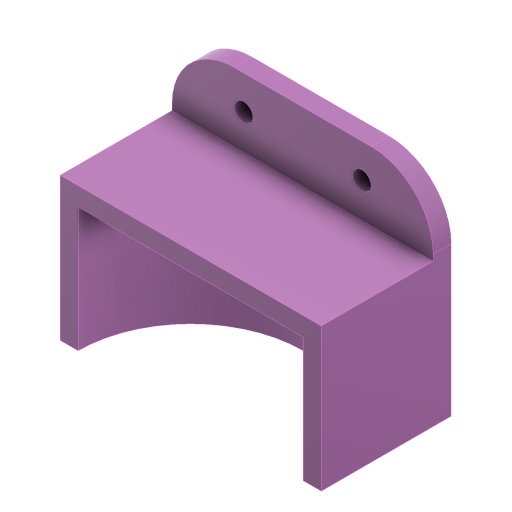
# Autodesk Inventor part: Держатель динамика
Saved by Autodesk Inventor 2024.1 (Build 281209000, 209)
## iProperties
Created: 2023-06-10
Part Number: Держатель динамика
Material: Типовые
Document SubType Name: Modeling
Designer: Admin
Density: 1 g/cm^3
Appearance: По умолчанию
Author: Admin
Autodesk Inventor part; units mm, degrees
ref_plane "YZ Plane" through (0, 0, 0) normal (1, 0, 0) x (0, 1, 0)
ref_plane "XZ Plane" through (0, 0, 0) normal (0, 1, 0) x (-1, 0, 0)
ref_plane "XY Plane" through (0, 0, 0) normal (0, 0, 1) x (1, 0, 0)
sketch "Эскиз1" plane through (0, 0, 0) normal (0, 0, 1) x (1, 0, 0)
  line L0 (-42, 24) -> (-42, 23)
  line L1 (-10, 34) -> (-32, 34)
  line L2 (-42, 23) -> (-42, 0)
  line L3 (0, 23) -> (-42, 23)
  line L4 (-42, 0) -> (0, 0)
  line L5 (-42, 23) -> (0, 23)
  line L6 (-27.8, 26.9412) -> (-30.5, 25.3823)
  line L7 (-30.5, 25.3823) -> (-33.2, 26.9412)
  circle A0 centre (-30.5, 28.5) radius 1.5
  line L8 (-27.8, 30.0588) -> (-27.8, 26.9412)
  line L9 (-33.2, 26.9412) -> (-33.2, 30.0588)
  arc A1 (-32, 34) -> (-42, 24) centre (-32, 24) ccw
  line L10 (-30.5, 31.6177) -> (-27.8, 30.0588)
  line L11 (-33.2, 30.0588) -> (-30.5, 31.6177)
  line L12 (-14.2, 26.9412) -> (-14.2, 30.0588)
  line L13 (-14.2, 30.0588) -> (-11.5, 31.6177)
  line L14 (-11.5, 25.3823) -> (-14.2, 26.9412)
  circle A2 centre (-11.5, 28.5) radius 1.5
  line L15 (-11.5, 31.6177) -> (-8.8, 30.0588)
  line L16 (-8.8, 30.0588) -> (-8.8, 26.9412)
  line L17 (-8.8, 26.9412) -> (-11.5, 25.3823)
  line L18 (0, 0) -> (0, 23)
  line L19 (0, 23) -> (0, 24)
  arc A3 (0, 24) -> (-10, 34) centre (-10, 24) ccw
  dimension "d0" = 23
  dimension "d1" = 5.4
  dimension "d2" = 10
  dimension "d4" = 4
  dimension "d5" = 4
  dimension "d7" = 4
  dimension "d8" = 10
  dimension "d9" = 10
  dimension "d10" = 42
  constraints: 41 end point, 5 coincident, 4 centre point, 4 perpendicular, 4 point on circle, 4 tangent, 3 vertical, 2 equal radius, 2 parallel, 1 collinear, 1 horizontal, 27 other
  measures "d0" distance of L2.end L0.end
  measures "d1" distance between parallel lines of L12 L16
  measures "d2" distance edge to line of A2 L19
  measures "d4" distance edge to line of A2 L1
  measures "d5" distance edge to line of A2 L3
  measures "d7" distance edge to line of A0 L1
  measures "d8" distance edge to line of A0 L0
  measures "d9" radius of A3
  measures "d10" distance of L2.end L18.start
extrude "Выдавливание1" add sketch "Эскиз1" along normal blind 21 contours L3 L18 L4 L2
sketch "Эскиз2" plane through (-42, 0, 0) normal (0, -1, 0) x (1, 0, 0)
  line L0 (0, 21) -> (42, 21) projected
  circle A0 centre (21, 21) radius 18.1
  point P0 (42, 0)
  point P1 (39.1, 21)
  point P2 (2.9, 21)
  constraints: 1 centre point, 1 midpoint, 1 other
extrude "Выдавливание2" cut sketch "Эскиз2" against normal blind 20 contours L0 A0 picked at (19.3763, 11.111)
extrude "Выдавливание3" add sketch "Эскиз1" along normal blind 3 contours A1 L1 A3 L19 L3 L0 | L6 L7 L9 L11 L10 L8 | L12 L13 L15 L16 L17 L14
chamfer "Фаска1" distance 0.3 distance2 0.1 5 edges at (0, 12, 0) (-2.9289, 31.0711, 0) (-21, 34, 0) (-39.0711, 31.0711, 0) (-21, 0, 0) measured on face at (-18.0106, 9.0325, 0)
